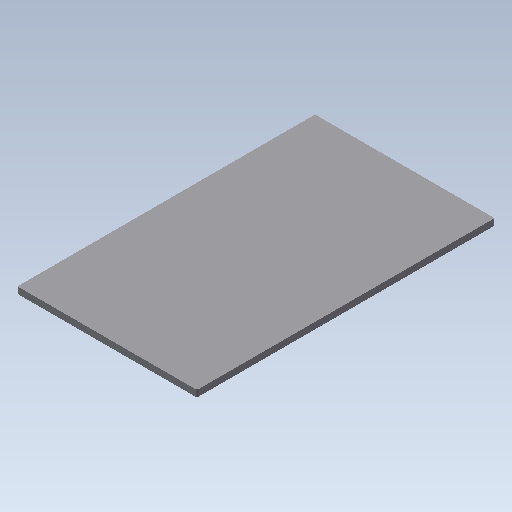
# Autodesk Inventor part: Standard
Saved by Autodesk Inventor 2020.3 (Build 243373000, 373)
## iProperties
RuleStatus: InUse
AfterDocSave0: file://Part Number Cleaner
Created: 2022-01-21
Material: Generic
Catalog Web Link: https://www.janelia.org/
Vendor: HHMI: JRC - jET
Document SubType Name: Modeling
Designer: solomone
Density: 1 g/cm^3
Appearance: Default
LAB/DEPT: A. LEE (LAB)
DESIGN DEPARTMENT: HHMI: JRC - jET
ALTERED ITEM PART NUMBER: N/A
ALTERED ITEM VENDOR: N/A
ALTERED ITEM DESCRIPTION: N/A
Title: Standard
Author: solomone
Revision Number: 0
Autodesk Inventor part; units mm, degrees
ref_plane "YZ Plane" through (0, 0, 0) normal (1, 0, 0) x (0, 1, 0)
ref_plane "XZ Plane" through (0, 0, 0) normal (0, 1, 0) x (-1, 0, 0)
ref_plane "XY Plane" through (0, 0, 0) normal (0, 0, 1) x (1, 0, 0)
sketch "Sketch1" plane through (0, 0, 0) normal (0, 1, 0) x (-1, 0, 0)
  line L0 (176.2125, -292.1) -> (-176.2125, -292.1)
  line L1 (-176.2125, -292.1) -> (-176.2125, 292.1)
  line L2 (-176.2125, 292.1) -> (176.2125, 292.1)
  line L3 (176.2125, 292.1) -> (176.2125, -292.1)
  point P0 (0, 0)
  dimension "d0" = 584.2
  dimension "d1" = 352.425
  dimension "d2" = 176.2125
  dimension "d3" = 292.1
  constraints: 8 end point, 2 parallel, 1 horizontal, 1 perpendicular
  measures "d0" distance between parallel lines of L2 L0
  measures "d1" distance between parallel lines of L1 L3
  measures "d2" distance from line of point (0, 0) L3
  measures "d3" distance from line of point (0, 0) L0
extrude "Extrusion1" add sketch "Sketch1" along normal blind 12.7
fillet "Fillet1" radius 3.175 4 edges at (-176.2125, 6.35, 292.1) (176.2125, 6.35, 292.1) (176.2125, 6.35, -292.1) (-176.2125, 6.35, -292.1)
equation "\"d2\" = 0.5 * d1"
equation "\"d3\" = 0.5 * d0"
body "Solid1"
